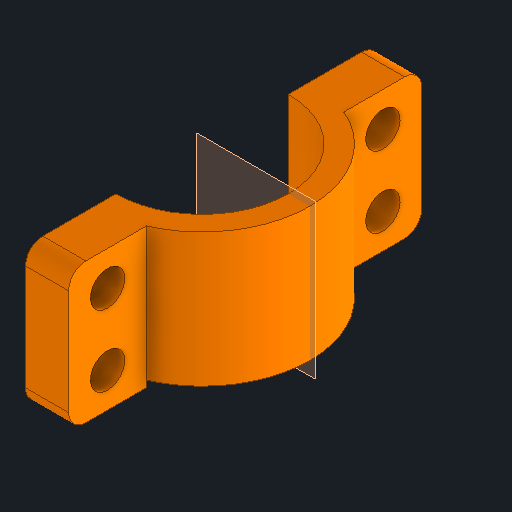
# Autodesk Inventor part: cup
Saved by Autodesk Inventor 2024 (Build 280153000, 153)
## iProperties
Created: 2023-05-13
Part Number: cup
Material: Типовые
Document SubType Name: Modeling
Designer: user
Density: 1 g/cm^3
Appearance: По умолчанию
Author: user
Autodesk Inventor part; units mm, degrees
ref_plane "YZ Plane" through (0, 0, 0) normal (1, 0, 0) x (0, 1, 0)
ref_plane "XZ Plane" through (0, 0, 0) normal (0, 1, 0) x (-1, 0, 0)
ref_plane "XY Plane" through (0, 0, 0) normal (0, 0, 1) x (1, 0, 0)
sketch "Эскиз1" plane through (0, 0, 0) normal (0, 0, 1) x (1, 0, 0)
  line L0 (-6.25, 10) -> (-6.25, 12.5) projected
  arc A0 (-6.25, -10) -> (-6.25, 10) centre (-6.25, 0) ccw projected
  line L1 (-6.25, -12.5) -> (-6.25, -10) projected
  arc A1 (-6.25, -12.5) -> (-6.25, 12.5) centre (-6.25, 0) ccw projected
  point P0 (0, 0)
ref_plane "РабПлоскость1" through (-18.75, -18.5, 15.5) normal (0, 0, 1) x (1, 0, 0)
extrude "Выдавливание1" add sketch "Эскиз1" along normal up to surface (15.5 mm away)
sketch "Эскиз2" plane through (-6.25, 0, 15.5) normal (0, 0, 1) x (1, 0, 0)
  line L0 (0, -18.5) -> (0, -20.5) projected
  line L1 (0, -18.5) -> (0, -10) projected
  line L2 (0, -20.5) -> (5, -20.5)
  line L3 (5, -20.5) -> (5, -11.4564)
  line L4 (0, -10) -> (0, -12.5) projected
  arc A0 (0, -12.5) -> (5, -11.4564) centre (0, 0) ccw
  arc A1 (0, -12.5) -> (0, 12.5) centre (0, 0) ccw projected
  line L5 (-5, -20.5) -> (0, -20.5) projected
  point P0 (6.25, 0)
  constraints: 4 end point, 2 point on circle, 1 centre point, 1 collinear, 1 concentric, 1 horizontal, 1 perpendicular
ref_plane "РабПлоскость2" through (-11.25, -18.5, -0.75) normal (0, 0, -1) x (0, 1, 0)
extrude "Выдавливание2" add sketch "Эскиз2" against normal up to surface (16.25 mm away)
sketch "Эскиз3" plane through (-6.25, -10, 0) normal (-1, 0, 0) x (0, 0, 1)
  circle A0 centre (11.5, -5.9782) radius 2 projected
  circle A1 centre (3.25, -5.9782) radius 2 projected
  point P0 (0, 10)
extrude "Выдавливание3" cut sketch "Эскиз3" against normal through all
fillet "Сопряжение1" radius 2 2 edges at (-3.75, -20.5, -0.75) (-3.75, -20.5, 15.5)
ref_plane "РабПлоскость3" through (3.75, 0, 15.5) normal (0, -1, 0) x (1, 0, 0)
mirror "Зеркальное отражение1" about plane through (3.75, 0, 15.5) normal (0, -1, 0) of "Сопряжение1", "Выдавливание3", "Выдавливание2"
